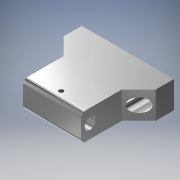
# Autodesk Inventor part: suporte_guia_central
Saved by Autodesk Inventor 2018 (Build 220112000, 112)
## iProperties
Created: 2018-05-16
Part Number: suporte_guia_central
Material: Alumínio 6061
Document SubType Name: Modeling
Designer: Usuario
Density: 2.7 g/cm^3
Appearance: Alumínio - Plano
Mass: 573.967 g
Surface Area: 310.294 cm^2
Volume: 212.58 cm^3
Author: Usuario
Autodesk Inventor part; units mm, degrees
ref_plane "YZ Plane" through (0, 0, 0) normal (1, 0, 0) x (0, 1, 0)
ref_plane "XZ Plane" through (0, 0, 0) normal (0, 1, 0) x (-1, 0, 0)
ref_plane "XY Plane" through (0, 0, 0) normal (0, 0, 1) x (1, 0, 0)
sketch "Esboço1" plane through (0, 0, 0) normal (0, 0, 1) x (1, 0, 0)
  line L0 (0, 36.3068) -> (0, -8.6932) construction
  circle A0 centre (0, -8.6932) radius 68 construction
  line L1 (0, 36.3068) -> (50.9804, 36.3068)
  line L2 (50.9804, 36.3068) -> (50.9804, 16.3068)
  line L3 (50.9804, 16.3068) -> (32.1355, -2.5381)
  line L4 (32.1355, -2.5381) -> (32.1355, -47.5381)
  line L5 (32.1355, -47.5381) -> (0, -47.5381)
  line L6 (0, -76.6932) -> (0, 59.3068) construction
  line L7 (0, 36.3068) -> (-50.9804, 36.3068)
  line L8 (-50.9804, 36.3068) -> (-50.9804, 16.3068)
  line L9 (-50.9804, 16.3068) -> (-32.1355, -2.5381)
  line L10 (-32.1355, -2.5381) -> (-32.1355, -47.5381)
  line L11 (-32.1355, -47.5381) -> (0, -47.5381)
  point P0 (0, 0)
  dimension "d1" = 45
  dimension "d2" = 136
  dimension "d3" = 20
  dimension "d4" = 135
  dimension "d5" = 45
  dimension "d7" = 50.9804
  constraints: 24 end point, 4 symmetric about line, 3 point on circle, 2 vertical, 1 centre point, 1 coincident, 1 perpendicular, 1 other
  measures "d1" distance of L0.start L0.end
  measures "d2" diameter of A0
  measures "d3" distance of L1.end L2.end
  measures "d4" angle of L2 L3
  measures "d5" distance of L3.end L4.end
  measures "d7" distance of L0.start L1.end
extrude "Extrusão1" add sketch "Esboço1" along normal mid plane 30
sketch "Esboço2" plane through (-32.1355, -47.5381, 15) normal (-1, 0, 0) x (0, 0, 1)
  line L0 (0, 0) -> (-30, 0) construction
  line L1 (-15, 0) -> (-15, 10) construction
  circle A0 centre (-15, 10) radius 6.075
  point P0 (-15, 47.5381)
  dimension "d10" = 10
  dimension "d11" = 12.15
  constraints: 2 end point, 1 centre point, 1 coincident, 1 midpoint, 1 vertical
  measures "d10" distance of L1.start L1.end
  measures "d11" diameter of A0
hole "Furo1" at (-32.1355, -37.5381, 0) direction (1, 0, 0) diameter 12.15 end through all
fillet "Arredondamento1" radius 5 2 edges at (0, -47.5381, 15) (0, -47.5381, -15)
sketch "Esboço3" plane through (0, 0, 15) normal (0, 0, 1) x (1, 0, 0)
  line L0 (0, 0) -> (0, -37.5381) construction
  constraints: 2 end point, 1 vertical
hole "Furo2" at (0, -37.5381, 15) direction (0, 0, -1) diameter 4.917 depth 10 tip angle 118 thread size "M6x1" class "6H" standard "ANSI Metric M Profile"
ref_plane "Plano de trabalho2" through (-32.1355, -2.5381, 0) normal (0, -1, 0) x (0, 0, -1)
sketch "Esboço6" plane through (-32.1355, -2.5381, 0) normal (0, -1, 0) x (0, 0, -1)
  line L0 (-15, 83.1159) -> (15, 83.1159) projected
  line L1 (0, 83.1159) -> (0, 73.8129) construction
  line L2 (0, -18.9836) -> (0, -9.9456)
  point P0 (0, 32.1355)
  dimension "d32" = 9.303
  dimension "d33" = 9.038
  constraints: 4 end point, 2 vertical, 1 midpoint
  measures "d32" distance of L1.start L1.end
  measures "d33" distance of L2.start L2.end
hole "Furo3" at (41.6774, -2.5381, 0) at (-42.0811, -2.5381, 0) direction (0, 1, 0) diameter 8.1 depth 44 tip angle 118 counterbore diameter 15 counterbore depth 30
